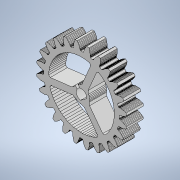
# Autodesk Inventor part: Деталь2
Saved by Autodesk Inventor 2020 (Build 240168000, 168)
## iProperties
Created: 2021-10-09
Part Number: Деталь2
Material: Типовые
Document SubType Name: Modeling
Designer: Антон
Density: 1 g/cm^3
Appearance: По умолчанию
Autodesk Inventor part; units mm, degrees
ref_plane "YZ Plane" through (0, 0, 0) normal (1, 0, 0) x (0, 1, 0)
ref_plane "XZ Plane" through (0, 0, 0) normal (0, 1, 0) x (-1, 0, 0)
ref_plane "XY Plane" through (0, 0, 0) normal (0, 0, 1) x (1, 0, 0)
sketch "a" plane through (0, 0, 0) normal (0, 0, 1) x (1, 0, 0)
  line L0 (2.444, 10.7729) -> (2.3647, 10.8798)
  line L1 (2.3647, 10.8798) -> (2.3022, 10.9131)
  line L2 (2.3022, 10.9131) -> (2.2426, 10.933)
  line L3 (2.2426, 10.933) -> (2.1279, 10.953)
  line L4 (2.1279, 10.953) -> (2.0158, 10.9612)
  line L5 (2.0158, 10.9612) -> (1.9071, 10.9524)
  line L6 (1.9071, 10.9524) -> (1.6861, 10.9538)
  line L7 (1.6861, 10.9538) -> (1.4617, 10.9732)
  line L8 (1.4617, 10.9732) -> (1.2349, 11.0072)
  line L9 (1.2349, 11.0072) -> (1.0063, 11.0542)
  line L10 (1.0063, 11.0542) -> (0.7762, 11.1131)
  line L11 (0.7762, 11.1131) -> (0.5451, 11.1834)
  line L12 (0.5451, 11.1834) -> (0.3132, 11.2645)
  line L13 (0.3132, 11.2645) -> (0.1389, 11.3323)
  line L14 (0.1389, 11.3323) -> (0.0609, 11.9767)
  line L15 (0.0609, 11.9767) -> (0.214, 12.084)
  line L16 (0.214, 12.084) -> (0.4199, 12.2181)
  line L17 (0.4199, 12.2181) -> (0.6276, 12.3415)
  line L18 (0.6276, 12.3415) -> (0.837, 12.4537)
  line L19 (0.837, 12.4537) -> (1.0478, 12.5538)
  line L20 (1.0478, 12.5538) -> (1.2599, 12.6409)
  line L21 (1.2599, 12.6409) -> (1.4731, 12.7133)
  line L22 (1.4731, 12.7133) -> (1.6875, 12.7674)
  line L23 (1.6875, 12.7674) -> (1.7951, 12.7847)
  line L24 (1.7951, 12.7847) -> (1.9021, 12.8194)
  line L25 (1.9021, 12.8194) -> (2.0087, 12.8663)
  line L26 (2.0087, 12.8663) -> (2.0617, 12.8998)
  line L27 (2.0617, 12.8998) -> (2.1145, 12.947)
  line L28 (2.1145, 12.947) -> (2.166, 13.0697)
  line L29 (2.166, 13.0697) -> (2.1721, 13.6527)
  line L30 (2.1721, 13.6527) -> (2.1232, 13.7765)
  line L31 (2.1232, 13.7765) -> (2.0714, 13.8248)
  line L32 (2.0714, 13.8248) -> (2.0191, 13.8595)
  line L33 (2.0191, 13.8595) -> (1.9135, 13.9085)
  line L34 (1.9135, 13.9085) -> (1.8073, 13.9455)
  line L35 (1.8073, 13.9455) -> (1.7, 13.965)
  line L36 (1.7, 13.965) -> (1.4869, 14.0236)
  line L37 (1.4869, 14.0236) -> (1.2752, 14.1004)
  line L38 (1.2752, 14.1004) -> (1.0649, 14.1919)
  line L39 (1.0649, 14.1919) -> (0.8563, 14.2965)
  line L40 (0.8563, 14.2965) -> (0.6493, 14.413)
  line L41 (0.6493, 14.413) -> (0.4442, 14.5407)
  line L42 (0.4442, 14.5407) -> (0.2412, 14.6791)
  line L43 (0.2412, 14.6791) -> (0.0903, 14.7897)
  line L44 (0.0903, 14.7897) -> (0.1818, 15.4322)
  line L45 (0.1818, 15.4322) -> (0.3575, 15.4963)
  line L46 (0.3575, 15.4963) -> (0.591, 15.5726)
  line L47 (0.591, 15.5726) -> (0.8236, 15.638)
  line L48 (0.8236, 15.638) -> (1.0549, 15.6921)
  line L49 (1.0549, 15.6921) -> (1.2845, 15.7343)
  line L50 (1.2845, 15.7343) -> (1.5119, 15.7636)
  line L51 (1.5119, 15.7636) -> (1.7366, 15.7782)
  line L52 (1.7366, 15.7782) -> (1.9576, 15.775)
  line L53 (1.9576, 15.775) -> (2.0661, 15.7639)
  line L54 (2.0661, 15.7639) -> (2.1784, 15.7697)
  line L55 (2.1784, 15.7697) -> (2.2935, 15.7874)
  line L56 (2.2935, 15.7874) -> (2.3534, 15.8061)
  line L57 (2.3534, 15.8061) -> (2.4166, 15.838)
  line L58 (2.4166, 15.838) -> (2.4981, 15.9432)
  line L59 (2.4981, 15.9432) -> (2.6549, 16.5048)
  line L60 (2.6549, 16.5048) -> (2.6397, 16.637)
  line L61 (2.6397, 16.637) -> (2.6022, 16.6971)
  line L62 (2.6022, 16.6971) -> (2.5606, 16.7441)
  line L63 (2.5606, 16.7441) -> (2.4713, 16.8188)
  line L64 (2.4713, 16.8188) -> (2.3782, 16.882)
  line L65 (2.3782, 16.882) -> (2.2797, 16.9286)
  line L66 (2.2797, 16.9286) -> (2.089, 17.0404)
  line L67 (2.089, 17.0404) -> (1.9044, 17.1693)
  line L68 (1.9044, 17.1693) -> (1.725, 17.3122)
  line L69 (1.725, 17.3122) -> (1.5505, 17.4672)
  line L70 (1.5505, 17.4672) -> (1.3807, 17.6333)
  line L71 (1.3807, 17.6333) -> (1.2157, 17.8097)
  line L72 (1.2157, 17.8097) -> (1.0554, 17.996)
  line L73 (1.0554, 17.996) -> (0.9383, 18.1418)
  line L74 (0.9383, 18.1418) -> (1.193, 18.7388)
  line L75 (1.193, 18.7388) -> (1.3792, 18.7552)
  line L76 (1.3792, 18.7552) -> (1.6246, 18.7684)
  line L77 (1.6246, 18.7684) -> (1.8662, 18.7714)
  line L78 (1.8662, 18.7714) -> (2.1036, 18.7639)
  line L79 (2.1036, 18.7639) -> (2.3362, 18.7452)
  line L80 (2.3362, 18.7452) -> (2.5635, 18.7146)
  line L81 (2.5635, 18.7146) -> (2.7843, 18.6706)
  line L82 (2.7843, 18.6706) -> (2.997, 18.6103)
  line L83 (2.997, 18.6103) -> (3.0989, 18.5715)
  line L84 (3.0989, 18.5715) -> (3.2088, 18.548)
  line L85 (3.2088, 18.548) -> (3.3246, 18.5353)
  line L86 (3.3246, 18.5353) -> (3.3873, 18.5378)
  line L87 (3.3873, 18.5378) -> (3.4566, 18.5523)
  line L88 (3.4566, 18.5523) -> (3.5626, 18.6328)
  line L89 (3.5626, 18.6328) -> (3.8594, 19.1347)
  line L90 (3.8594, 19.1347) -> (3.8789, 19.2664)
  line L91 (3.8789, 19.2664) -> (3.8582, 19.3341)
  line L92 (3.8582, 19.3341) -> (3.8302, 19.3902)
  line L93 (3.8302, 19.3902) -> (3.7633, 19.4855)
  line L94 (3.7633, 19.4855) -> (3.6898, 19.5707)
  line L95 (3.6898, 19.5707) -> (3.6067, 19.6412)
  line L96 (3.6067, 19.6412) -> (3.4514, 19.7985)
  line L97 (3.4514, 19.7985) -> (3.3065, 19.9709)
  line L98 (3.3065, 19.9709) -> (3.1701, 20.1552)
  line L99 (3.1701, 20.1552) -> (3.0417, 20.3501)
  line L100 (3.0417, 20.3501) -> (2.9207, 20.5545)
  line L101 (2.9207, 20.5545) -> (2.807, 20.7677)
  line L102 (2.807, 20.7677) -> (2.7003, 20.989)
  line L103 (2.7003, 20.989) -> (2.625, 21.1602)
  line L104 (2.625, 21.1602) -> (3.0255, 21.671)
  line L105 (3.0255, 21.671) -> (3.2096, 21.6386)
  line L106 (3.2096, 21.6386) -> (3.4501, 21.5878)
  line L107 (3.4501, 21.5878) -> (3.6842, 21.5282)
  line L108 (3.6842, 21.5282) -> (3.9115, 21.4595)
  line L109 (3.9115, 21.4595) -> (4.1314, 21.3812)
  line L110 (4.1314, 21.3812) -> (4.343, 21.2929)
  line L111 (4.343, 21.2929) -> (4.545, 21.1932)
  line L112 (4.545, 21.1932) -> (4.7348, 21.0799)
  line L113 (4.7348, 21.0799) -> (4.8231, 21.016)
  line L114 (4.8231, 21.016) -> (4.9233, 20.965)
  line L115 (4.9233, 20.965) -> (5.0318, 20.9227)
  line L116 (5.0318, 20.9227) -> (5.093, 20.9089)
  line L117 (5.093, 20.9089) -> (5.1637, 20.9049)
  line L118 (5.1637, 20.9049) -> (5.287, 20.9553)
  line L119 (5.287, 20.9553) -> (5.7035, 21.3632)
  line L120 (5.7035, 21.3632) -> (5.7565, 21.4854)
  line L121 (5.7565, 21.4854) -> (5.754, 21.5561)
  line L122 (5.754, 21.5561) -> (5.7415, 21.6176)
  line L123 (5.7415, 21.6176) -> (5.7015, 21.727)
  line L124 (5.7015, 21.727) -> (5.6525, 21.8283)
  line L125 (5.6525, 21.8283) -> (5.5905, 21.9179)
  line L126 (5.5905, 21.9179) -> (5.4812, 22.1101)
  line L127 (5.4812, 22.1101) -> (5.3858, 22.314)
  line L128 (5.3858, 22.314) -> (5.3019, 22.5274)
  line L129 (5.3019, 22.5274) -> (5.2283, 22.7489)
  line L130 (5.2283, 22.7489) -> (5.1643, 22.9777)
  line L131 (5.1643, 22.9777) -> (5.1096, 23.213)
  line L132 (5.1096, 23.213) -> (5.0639, 23.4544)
  line L133 (5.0639, 23.4544) -> (5.0354, 23.6392)
  line L134 (5.0354, 23.6392) -> (5.5544, 24.0289)
  line L135 (5.5544, 24.0289) -> (5.724, 23.95)
  line L136 (5.724, 23.95) -> (5.943, 23.8388)
  line L137 (5.943, 23.8388) -> (6.1538, 23.7206)
  line L138 (6.1538, 23.7206) -> (6.3556, 23.5953)
  line L139 (6.3556, 23.5953) -> (6.5477, 23.4628)
  line L140 (6.5477, 23.4628) -> (6.7292, 23.3227)
  line L141 (6.7292, 23.3227) -> (6.8985, 23.1742)
  line L142 (6.8985, 23.1742) -> (7.0525, 23.0156)
  line L143 (7.0525, 23.0156) -> (7.1213, 22.9311)
  line L144 (7.1213, 22.9311) -> (7.2049, 22.8558)
  line L145 (7.2049, 22.8558) -> (7.2988, 22.7869)
  line L146 (7.2988, 22.7869) -> (7.3543, 22.7577)
  line L147 (7.3543, 22.7577) -> (7.4216, 22.7356)
  line L148 (7.4216, 22.7356) -> (7.5536, 22.7523)
  line L149 (7.5536, 22.7523) -> (8.0616, 23.0386)
  line L150 (8.0616, 23.0386) -> (8.1443, 23.1428)
  line L151 (8.1443, 23.1428) -> (8.1603, 23.2118)
  line L152 (8.1603, 23.2118) -> (8.1641, 23.2745)
  line L153 (8.1641, 23.2745) -> (8.1538, 23.3905)
  line L154 (8.1538, 23.3905) -> (8.1327, 23.5009)
  line L155 (8.1327, 23.5009) -> (8.096, 23.6036)
  line L156 (8.096, 23.6036) -> (8.0402, 23.8175)
  line L157 (8.0402, 23.8175) -> (8.0008, 24.0392)
  line L158 (8.0008, 24.0392) -> (7.975, 24.267)
  line L159 (7.975, 24.267) -> (7.9612, 24.5)
  line L160 (7.9612, 24.5) -> (7.9586, 24.7375)
  line L161 (7.9586, 24.7375) -> (7.9666, 24.979)
  line L162 (7.9666, 24.979) -> (7.985, 25.224)
  line L163 (7.985, 25.224) -> (8.0053, 25.4099)
  line L164 (8.0053, 25.4099) -> (8.6075, 25.652)
  line L165 (8.6075, 25.652) -> (8.7508, 25.5319)
  line L166 (8.7508, 25.5319) -> (8.9337, 25.3677)
  line L167 (8.9337, 25.3677) -> (9.1066, 25.199)
  line L168 (9.1066, 25.199) -> (9.2691, 25.0258)
  line L169 (9.2691, 25.0258) -> (9.4205, 24.8481)
  line L170 (9.4205, 24.8481) -> (9.5595, 24.6658)
  line L171 (9.5595, 24.6658) -> (9.6846, 24.4785)
  line L172 (9.6846, 24.4785) -> (9.7923, 24.2855)
  line L173 (9.7923, 24.2855) -> (9.8369, 24.186)
  line L174 (9.8369, 24.186) -> (9.8981, 24.0917)
  line L175 (9.8981, 24.0917) -> (9.9709, 24.0008)
  line L176 (9.9709, 24.0008) -> (10.0171, 23.9582)
  line L177 (10.0171, 23.9582) -> (10.0763, 23.9195)
  line L178 (10.0763, 23.9195) -> (10.2082, 23.9015)
  line L179 (10.2082, 23.9015) -> (10.7729, 24.0465)
  line L180 (10.7729, 24.0465) -> (10.8798, 24.1258)
  line L181 (10.8798, 24.1258) -> (10.9131, 24.1883)
  line L182 (10.9131, 24.1883) -> (10.933, 24.2478)
  line L183 (10.933, 24.2478) -> (10.953, 24.3626)
  line L184 (10.953, 24.3626) -> (10.9612, 24.4747)
  line L185 (10.9612, 24.4747) -> (10.9524, 24.5833)
  line L186 (10.9524, 24.5833) -> (10.9538, 24.8044)
  line L187 (10.9538, 24.8044) -> (10.9732, 25.0287)
  line L188 (10.9732, 25.0287) -> (11.0072, 25.2555)
  line L189 (11.0072, 25.2555) -> (11.0542, 25.4842)
  line L190 (11.0542, 25.4842) -> (11.1131, 25.7142)
  line L191 (11.1131, 25.7142) -> (11.1834, 25.9454)
  line L192 (11.1834, 25.9454) -> (11.2645, 26.1773)
  line L193 (11.2645, 26.1773) -> (11.3323, 26.3516)
  line L194 (11.3323, 26.3516) -> (11.9767, 26.4296)
  line L195 (11.9767, 26.4296) -> (12.084, 26.2765)
  line L196 (12.084, 26.2765) -> (12.2181, 26.0706)
  line L197 (12.2181, 26.0706) -> (12.3415, 25.8629)
  line L198 (12.3415, 25.8629) -> (12.4537, 25.6535)
  line L199 (12.4537, 25.6535) -> (12.5538, 25.4427)
  line L200 (12.5538, 25.4427) -> (12.6409, 25.2306)
  line L201 (12.6409, 25.2306) -> (12.7133, 25.0173)
  line L202 (12.7133, 25.0173) -> (12.7674, 24.803)
  line L203 (12.7674, 24.803) -> (12.7847, 24.6954)
  line L204 (12.7847, 24.6954) -> (12.8194, 24.5884)
  line L205 (12.8194, 24.5884) -> (12.8663, 24.4818)
  line L206 (12.8663, 24.4818) -> (12.8998, 24.4287)
  line L207 (12.8998, 24.4287) -> (12.947, 24.3759)
  line L208 (12.947, 24.3759) -> (13.0697, 24.3244)
  line L209 (13.0697, 24.3244) -> (13.6527, 24.3183)
  line L210 (13.6527, 24.3183) -> (13.7765, 24.3673)
  line L211 (13.7765, 24.3673) -> (13.8248, 24.419)
  line L212 (13.8248, 24.419) -> (13.8595, 24.4714)
  line L213 (13.8595, 24.4714) -> (13.9085, 24.577)
  line L214 (13.9085, 24.577) -> (13.9455, 24.6832)
  line L215 (13.9455, 24.6832) -> (13.965, 24.7904)
  line L216 (13.965, 24.7904) -> (14.0236, 25.0036)
  line L217 (14.0236, 25.0036) -> (14.1004, 25.2153)
  line L218 (14.1004, 25.2153) -> (14.1919, 25.4255)
  line L219 (14.1919, 25.4255) -> (14.2965, 25.6342)
  line L220 (14.2965, 25.6342) -> (14.413, 25.8412)
  line L221 (14.413, 25.8412) -> (14.5407, 26.0463)
  line L222 (14.5407, 26.0463) -> (14.6791, 26.2493)
  line L223 (14.6791, 26.2493) -> (14.7897, 26.4001)
  line L224 (14.7897, 26.4001) -> (15.4322, 26.3087)
  line L225 (15.4322, 26.3087) -> (15.4963, 26.133)
  line L226 (15.4963, 26.133) -> (15.5726, 25.8994)
  line L227 (15.5726, 25.8994) -> (15.638, 25.6668)
  line L228 (15.638, 25.6668) -> (15.6921, 25.4356)
  line L229 (15.6921, 25.4356) -> (15.7343, 25.206)
  line L230 (15.7343, 25.206) -> (15.7636, 24.9786)
  line L231 (15.7636, 24.9786) -> (15.7782, 24.7539)
  line L232 (15.7782, 24.7539) -> (15.775, 24.5329)
  line L233 (15.775, 24.5329) -> (15.7639, 24.4244)
  line L234 (15.7639, 24.4244) -> (15.7697, 24.3121)
  line L235 (15.7697, 24.3121) -> (15.7874, 24.197)
  line L236 (15.7874, 24.197) -> (15.8061, 24.1371)
  line L237 (15.8061, 24.1371) -> (15.838, 24.0739)
  line L238 (15.838, 24.0739) -> (15.9432, 23.9924)
  line L239 (15.9432, 23.9924) -> (16.5048, 23.8356)
  line L240 (16.5048, 23.8356) -> (16.637, 23.8508)
  line L241 (16.637, 23.8508) -> (16.6971, 23.8883)
  line L242 (16.6971, 23.8883) -> (16.7441, 23.9299)
  line L243 (16.7441, 23.9299) -> (16.8188, 24.0192)
  line L244 (16.8188, 24.0192) -> (16.882, 24.1122)
  line L245 (16.882, 24.1122) -> (16.9286, 24.2108)
  line L246 (16.9286, 24.2108) -> (17.0404, 24.4015)
  line L247 (17.0404, 24.4015) -> (17.1693, 24.5861)
  line L248 (17.1693, 24.5861) -> (17.3122, 24.7655)
  line L249 (17.3122, 24.7655) -> (17.4672, 24.94)
  line L250 (17.4672, 24.94) -> (17.6333, 25.1097)
  line L251 (17.6333, 25.1097) -> (17.8097, 25.2748)
  line L252 (17.8097, 25.2748) -> (17.996, 25.4351)
  line L253 (17.996, 25.4351) -> (18.1418, 25.5522)
  line L254 (18.1418, 25.5522) -> (18.7388, 25.2975)
  line L255 (18.7388, 25.2975) -> (18.7552, 25.1112)
  line L256 (18.7552, 25.1112) -> (18.7684, 24.8659)
  line L257 (18.7684, 24.8659) -> (18.7714, 24.6243)
  line L258 (18.7714, 24.6243) -> (18.7639, 24.3869)
  line L259 (18.7639, 24.3869) -> (18.7452, 24.1542)
  line L260 (18.7452, 24.1542) -> (18.7146, 23.927)
  line L261 (18.7146, 23.927) -> (18.6706, 23.7061)
  line L262 (18.6706, 23.7061) -> (18.6103, 23.4935)
  line L263 (18.6103, 23.4935) -> (18.5715, 23.3916)
  line L264 (18.5715, 23.3916) -> (18.548, 23.2816)
  line L265 (18.548, 23.2816) -> (18.5353, 23.1659)
  line L266 (18.5353, 23.1659) -> (18.5378, 23.1031)
  line L267 (18.5378, 23.1031) -> (18.5523, 23.0338)
  line L268 (18.5523, 23.0338) -> (18.6328, 22.9279)
  line L269 (18.6328, 22.9279) -> (19.1347, 22.6311)
  line L270 (19.1347, 22.6311) -> (19.2664, 22.6115)
  line L271 (19.2664, 22.6115) -> (19.3341, 22.6322)
  line L272 (19.3341, 22.6322) -> (19.3902, 22.6603)
  line L273 (19.3902, 22.6603) -> (19.4855, 22.7272)
  line L274 (19.4855, 22.7272) -> (19.5707, 22.8007)
  line L275 (19.5707, 22.8007) -> (19.6412, 22.8838)
  line L276 (19.6412, 22.8838) -> (19.7985, 23.0391)
  line L277 (19.7985, 23.0391) -> (19.9709, 23.184)
  line L278 (19.9709, 23.184) -> (20.1552, 23.3203)
  line L279 (20.1552, 23.3203) -> (20.3501, 23.4488)
  line L280 (20.3501, 23.4488) -> (20.5545, 23.5698)
  line L281 (20.5545, 23.5698) -> (20.7677, 23.6835)
  line L282 (20.7677, 23.6835) -> (20.989, 23.7902)
  line L283 (20.989, 23.7902) -> (21.1602, 23.8655)
  line L284 (21.1602, 23.8655) -> (21.671, 23.465)
  line L285 (21.671, 23.465) -> (21.6386, 23.2808)
  line L286 (21.6386, 23.2808) -> (21.5878, 23.0404)
  line L287 (21.5878, 23.0404) -> (21.5282, 22.8063)
  line L288 (21.5282, 22.8063) -> (21.4595, 22.5789)
  line L289 (21.4595, 22.5789) -> (21.3812, 22.359)
  line L290 (21.3812, 22.359) -> (21.2929, 22.1475)
  line L291 (21.2929, 22.1475) -> (21.1932, 21.9455)
  line L292 (21.1932, 21.9455) -> (21.0799, 21.7557)
  line L293 (21.0799, 21.7557) -> (21.016, 21.6674)
  line L294 (21.016, 21.6674) -> (20.965, 21.5672)
  line L295 (20.965, 21.5672) -> (20.9227, 21.4587)
  line L296 (20.9227, 21.4587) -> (20.9089, 21.3974)
  line L297 (20.9089, 21.3974) -> (20.9049, 21.3267)
  line L298 (20.9049, 21.3267) -> (20.9553, 21.2035)
  line L299 (20.9553, 21.2035) -> (21.3632, 20.7869)
  line L300 (21.3632, 20.7869) -> (21.4854, 20.734)
  line L301 (21.4854, 20.734) -> (21.5561, 20.7365)
  line L302 (21.5561, 20.7365) -> (21.6176, 20.749)
  line L303 (21.6176, 20.749) -> (21.727, 20.789)
  line L304 (21.727, 20.789) -> (21.8283, 20.838)
  line L305 (21.8283, 20.838) -> (21.9179, 20.9)
  line L306 (21.9179, 20.9) -> (22.1101, 21.0093)
  line L307 (22.1101, 21.0093) -> (22.314, 21.1046)
  line L308 (22.314, 21.1046) -> (22.5274, 21.1886)
  line L309 (22.5274, 21.1886) -> (22.7489, 21.2622)
  line L310 (22.7489, 21.2622) -> (22.9777, 21.3262)
  line L311 (22.9777, 21.3262) -> (23.213, 21.3809)
  line L312 (23.213, 21.3809) -> (23.4544, 21.4266)
  line L313 (23.4544, 21.4266) -> (23.6392, 21.4551)
  line L314 (23.6392, 21.4551) -> (24.0289, 20.936)
  line L315 (24.0289, 20.936) -> (23.95, 20.7665)
  line L316 (23.95, 20.7665) -> (23.8388, 20.5474)
  line L317 (23.8388, 20.5474) -> (23.7206, 20.3367)
  line L318 (23.7206, 20.3367) -> (23.5953, 20.1349)
  line L319 (23.5953, 20.1349) -> (23.4628, 19.9427)
  line L320 (23.4628, 19.9427) -> (23.3227, 19.7612)
  line L321 (23.3227, 19.7612) -> (23.1742, 19.592)
  line L322 (23.1742, 19.592) -> (23.0156, 19.4379)
  line L323 (23.0156, 19.4379) -> (22.9311, 19.3692)
  line L324 (22.9311, 19.3692) -> (22.8558, 19.2856)
  line L325 (22.8558, 19.2856) -> (22.7869, 19.1917)
  line L326 (22.7869, 19.1917) -> (22.7577, 19.1361)
  line L327 (22.7577, 19.1361) -> (22.7356, 19.0689)
  line L328 (22.7356, 19.0689) -> (22.7523, 18.9368)
  line L329 (22.7523, 18.9368) -> (23.0386, 18.4289)
  line L330 (23.0386, 18.4289) -> (23.1428, 18.3461)
  line L331 (23.1428, 18.3461) -> (23.2118, 18.3302)
  line L332 (23.2118, 18.3302) -> (23.2745, 18.3264)
  line L333 (23.2745, 18.3264) -> (23.3905, 18.3367)
  line L334 (23.3905, 18.3367) -> (23.5009, 18.3578)
  line L335 (23.5009, 18.3578) -> (23.6036, 18.3945)
  line L336 (23.6036, 18.3945) -> (23.8175, 18.4503)
  line L337 (23.8175, 18.4503) -> (24.0392, 18.4897)
  line L338 (24.0392, 18.4897) -> (24.267, 18.5155)
  line L339 (24.267, 18.5155) -> (24.5, 18.5293)
  line L340 (24.5, 18.5293) -> (24.7375, 18.5319)
  line L341 (24.7375, 18.5319) -> (24.979, 18.5238)
  line L342 (24.979, 18.5238) -> (25.224, 18.5055)
  line L343 (25.224, 18.5055) -> (25.4099, 18.4852)
  line L344 (25.4099, 18.4852) -> (25.652, 17.883)
  line L345 (25.652, 17.883) -> (25.5319, 17.7396)
  line L346 (25.5319, 17.7396) -> (25.3677, 17.5568)
  line L347 (25.3677, 17.5568) -> (25.199, 17.3839)
  line L348 (25.199, 17.3839) -> (25.0258, 17.2213)
  line L349 (25.0258, 17.2213) -> (24.8481, 17.07)
  line L350 (24.8481, 17.07) -> (24.6658, 16.931)
  line L351 (24.6658, 16.931) -> (24.4785, 16.8059)
  line L352 (24.4785, 16.8059) -> (24.2855, 16.6982)
  line L353 (24.2855, 16.6982) -> (24.186, 16.6536)
  line L354 (24.186, 16.6536) -> (24.0917, 16.5924)
  line L355 (24.0917, 16.5924) -> (24.0008, 16.5195)
  line L356 (24.0008, 16.5195) -> (23.9582, 16.4734)
  line L357 (23.9582, 16.4734) -> (23.9195, 16.4142)
  line L358 (23.9195, 16.4142) -> (23.9015, 16.2823)
  line L359 (23.9015, 16.2823) -> (24.0465, 15.7175)
  line L360 (24.0465, 15.7175) -> (24.1258, 15.6106)
  line L361 (24.1258, 15.6106) -> (24.1883, 15.5774)
  line L362 (24.1883, 15.5774) -> (24.2478, 15.5575)
  line L363 (24.2478, 15.5575) -> (24.3626, 15.5374)
  line L364 (24.3626, 15.5374) -> (24.4747, 15.5292)
  line L365 (24.4747, 15.5292) -> (24.5833, 15.5381)
  line L366 (24.5833, 15.5381) -> (24.8044, 15.5367)
  line L367 (24.8044, 15.5367) -> (25.0287, 15.5173)
  line L368 (25.0287, 15.5173) -> (25.2555, 15.4833)
  line L369 (25.2555, 15.4833) -> (25.4842, 15.4363)
  line L370 (25.4842, 15.4363) -> (25.7142, 15.3773)
  line L371 (25.7142, 15.3773) -> (25.9454, 15.307)
  line L372 (25.9454, 15.307) -> (26.1773, 15.2259)
  line L373 (26.1773, 15.2259) -> (26.3516, 15.1582)
  line L374 (26.3516, 15.1582) -> (26.4296, 14.5138)
  line L375 (26.4296, 14.5138) -> (26.2765, 14.4065)
  line L376 (26.2765, 14.4065) -> (26.0706, 14.2724)
  line L377 (26.0706, 14.2724) -> (25.8629, 14.149)
  line L378 (25.8629, 14.149) -> (25.6535, 14.0368)
  line L379 (25.6535, 14.0368) -> (25.4427, 13.9366)
  line L380 (25.4427, 13.9366) -> (25.2306, 13.8495)
  line L381 (25.2306, 13.8495) -> (25.0173, 13.7772)
  line L382 (25.0173, 13.7772) -> (24.803, 13.7231)
  line L383 (24.803, 13.7231) -> (24.6954, 13.7058)
  line L384 (24.6954, 13.7058) -> (24.5884, 13.6711)
  line L385 (24.5884, 13.6711) -> (24.4818, 13.6242)
  line L386 (24.4818, 13.6242) -> (24.4287, 13.5907)
  line L387 (24.4287, 13.5907) -> (24.3759, 13.5435)
  line L388 (24.3759, 13.5435) -> (24.3244, 13.4208)
  line L389 (24.3244, 13.4208) -> (24.3183, 12.8377)
  line L390 (24.3183, 12.8377) -> (24.3673, 12.7139)
  line L391 (24.3673, 12.7139) -> (24.419, 12.6657)
  line L392 (24.419, 12.6657) -> (24.4714, 12.631)
  line L393 (24.4714, 12.631) -> (24.577, 12.5819)
  line L394 (24.577, 12.5819) -> (24.6832, 12.545)
  line L395 (24.6832, 12.545) -> (24.7904, 12.5254)
  line L396 (24.7904, 12.5254) -> (25.0036, 12.4669)
  line L397 (25.0036, 12.4669) -> (25.2153, 12.3901)
  line L398 (25.2153, 12.3901) -> (25.4255, 12.2985)
  line L399 (25.4255, 12.2985) -> (25.6342, 12.194)
  line L400 (25.6342, 12.194) -> (25.8412, 12.0775)
  line L401 (25.8412, 12.0775) -> (26.0463, 11.9498)
  line L402 (26.0463, 11.9498) -> (26.2493, 11.8114)
  line L403 (26.2493, 11.8114) -> (26.4001, 11.7008)
  line L404 (26.4001, 11.7008) -> (26.3087, 11.0582)
  line L405 (26.3087, 11.0582) -> (26.133, 10.9942)
  line L406 (26.133, 10.9942) -> (25.8994, 10.9179)
  line L407 (25.8994, 10.9179) -> (25.6668, 10.8525)
  line L408 (25.6668, 10.8525) -> (25.4356, 10.7983)
  line L409 (25.4356, 10.7983) -> (25.206, 10.7561)
  line L410 (25.206, 10.7561) -> (24.9786, 10.7269)
  line L411 (24.9786, 10.7269) -> (24.7539, 10.7122)
  line L412 (24.7539, 10.7122) -> (24.5329, 10.7154)
  line L413 (24.5329, 10.7154) -> (24.4244, 10.7266)
  line L414 (24.4244, 10.7266) -> (24.3121, 10.7207)
  line L415 (24.3121, 10.7207) -> (24.197, 10.7031)
  line L416 (24.197, 10.7031) -> (24.1371, 10.6844)
  line L417 (24.1371, 10.6844) -> (24.0739, 10.6525)
  line L418 (24.0739, 10.6525) -> (23.9924, 10.5473)
  line L419 (23.9924, 10.5473) -> (23.8356, 9.9857)
  line L420 (23.8356, 9.9857) -> (23.8508, 9.8535)
  line L421 (23.8508, 9.8535) -> (23.8883, 9.7934)
  line L422 (23.8883, 9.7934) -> (23.9299, 9.7464)
  line L423 (23.9299, 9.7464) -> (24.0192, 9.6717)
  line L424 (24.0192, 9.6717) -> (24.1122, 9.6085)
  line L425 (24.1122, 9.6085) -> (24.2108, 9.5618)
  line L426 (24.2108, 9.5618) -> (24.4015, 9.4501)
  line L427 (24.4015, 9.4501) -> (24.5861, 9.3211)
  line L428 (24.5861, 9.3211) -> (24.7655, 9.1783)
  line L429 (24.7655, 9.1783) -> (24.94, 9.0233)
  line L430 (24.94, 9.0233) -> (25.1097, 8.8572)
  line L431 (25.1097, 8.8572) -> (25.2748, 8.6807)
  line L432 (25.2748, 8.6807) -> (25.4351, 8.4945)
  line L433 (25.4351, 8.4945) -> (25.5522, 8.3487)
  line L434 (25.5522, 8.3487) -> (25.2975, 7.7517)
  line L435 (25.2975, 7.7517) -> (25.1112, 7.7353)
  line L436 (25.1112, 7.7353) -> (24.8659, 7.7221)
  line L437 (24.8659, 7.7221) -> (24.6243, 7.7191)
  line L438 (24.6243, 7.7191) -> (24.3869, 7.7266)
  line L439 (24.3869, 7.7266) -> (24.1542, 7.7453)
  line L440 (24.1542, 7.7453) -> (23.927, 7.7759)
  line L441 (23.927, 7.7759) -> (23.7061, 7.8199)
  line L442 (23.7061, 7.8199) -> (23.4935, 7.8802)
  line L443 (23.4935, 7.8802) -> (23.3916, 7.919)
  line L444 (23.3916, 7.919) -> (23.2816, 7.9424)
  line L445 (23.2816, 7.9424) -> (23.1659, 7.9552)
  line L446 (23.1659, 7.9552) -> (23.1031, 7.9527)
  line L447 (23.1031, 7.9527) -> (23.0338, 7.9382)
  line L448 (23.0338, 7.9382) -> (22.9279, 7.8576)
  line L449 (22.9279, 7.8576) -> (22.6311, 7.3558)
  line L450 (22.6311, 7.3558) -> (22.6115, 7.2241)
  line L451 (22.6115, 7.2241) -> (22.6322, 7.1564)
  line L452 (22.6322, 7.1564) -> (22.6603, 7.1002)
  line L453 (22.6603, 7.1002) -> (22.7272, 7.0049)
  line L454 (22.7272, 7.0049) -> (22.8007, 6.9198)
  line L455 (22.8007, 6.9198) -> (22.8838, 6.8493)
  line L456 (22.8838, 6.8493) -> (23.0391, 6.692)
  line L457 (23.0391, 6.692) -> (23.184, 6.5196)
  line L458 (23.184, 6.5196) -> (23.3203, 6.3352)
  line L459 (23.3203, 6.3352) -> (23.4488, 6.1403)
  line L460 (23.4488, 6.1403) -> (23.5698, 5.936)
  line L461 (23.5698, 5.936) -> (23.6835, 5.7228)
  line L462 (23.6835, 5.7228) -> (23.7902, 5.5014)
  line L463 (23.7902, 5.5014) -> (23.8655, 5.3303)
  line L464 (23.8655, 5.3303) -> (23.465, 4.8195)
  line L465 (23.465, 4.8195) -> (23.2808, 4.8519)
  line L466 (23.2808, 4.8519) -> (23.0404, 4.9026)
  line L467 (23.0404, 4.9026) -> (22.8063, 4.9623)
  line L468 (22.8063, 4.9623) -> (22.5789, 5.031)
  line L469 (22.5789, 5.031) -> (22.359, 5.1092)
  line L470 (22.359, 5.1092) -> (22.1475, 5.1976)
  line L471 (22.1475, 5.1976) -> (21.9455, 5.2973)
  line L472 (21.9455, 5.2973) -> (21.7557, 5.4105)
  line L473 (21.7557, 5.4105) -> (21.6674, 5.4744)
  line L474 (21.6674, 5.4744) -> (21.5672, 5.5255)
  line L475 (21.5672, 5.5255) -> (21.4587, 5.5678)
  line L476 (21.4587, 5.5678) -> (21.3974, 5.5816)
  line L477 (21.3974, 5.5816) -> (21.3267, 5.5855)
  line L478 (21.3267, 5.5855) -> (21.2035, 5.5352)
  line L479 (21.2035, 5.5352) -> (20.7869, 5.1272)
  line L480 (20.7869, 5.1272) -> (20.734, 5.0051)
  line L481 (20.734, 5.0051) -> (20.7365, 4.9343)
  line L482 (20.7365, 4.9343) -> (20.749, 4.8728)
  line L483 (20.749, 4.8728) -> (20.789, 4.7634)
  line L484 (20.789, 4.7634) -> (20.838, 4.6622)
  line L485 (20.838, 4.6622) -> (20.9, 4.5726)
  line L486 (20.9, 4.5726) -> (21.0093, 4.3804)
  line L487 (21.0093, 4.3804) -> (21.1046, 4.1764)
  line L488 (21.1046, 4.1764) -> (21.1886, 3.963)
  line L489 (21.1886, 3.963) -> (21.2622, 3.7416)
  line L490 (21.2622, 3.7416) -> (21.3262, 3.5128)
  line L491 (21.3262, 3.5128) -> (21.3809, 3.2775)
  line L492 (21.3809, 3.2775) -> (21.4266, 3.0361)
  line L493 (21.4266, 3.0361) -> (21.4551, 2.8513)
  line L494 (21.4551, 2.8513) -> (20.936, 2.4615)
  line L495 (20.936, 2.4615) -> (20.7665, 2.5405)
  line L496 (20.7665, 2.5405) -> (20.5474, 2.6517)
  line L497 (20.5474, 2.6517) -> (20.3367, 2.7699)
  line L498 (20.3367, 2.7699) -> (20.1349, 2.8951)
  line L499 (20.1349, 2.8951) -> (19.9427, 3.0276)
  line L500 (19.9427, 3.0276) -> (19.7612, 3.1678)
  line L501 (19.7612, 3.1678) -> (19.592, 3.3163)
  line L502 (19.592, 3.3163) -> (19.4379, 3.4749)
  line L503 (19.4379, 3.4749) -> (19.3692, 3.5594)
  line L504 (19.3692, 3.5594) -> (19.2856, 3.6347)
  line L505 (19.2856, 3.6347) -> (19.1917, 3.7036)
  line L506 (19.1917, 3.7036) -> (19.1361, 3.7328)
  line L507 (19.1361, 3.7328) -> (19.0689, 3.7549)
  line L508 (19.0689, 3.7549) -> (18.9368, 3.7381)
  line L509 (18.9368, 3.7381) -> (18.4289, 3.4519)
  line L510 (18.4289, 3.4519) -> (18.3461, 3.3476)
  line L511 (18.3461, 3.3476) -> (18.3302, 3.2787)
  line L512 (18.3302, 3.2787) -> (18.3264, 3.216)
  line L513 (18.3264, 3.216) -> (18.3367, 3.1)
  line L514 (18.3367, 3.1) -> (18.3578, 2.9895)
  line L515 (18.3578, 2.9895) -> (18.3945, 2.8869)
  line L516 (18.3945, 2.8869) -> (18.4503, 2.673)
  line L517 (18.4503, 2.673) -> (18.4897, 2.4513)
  line L518 (18.4897, 2.4513) -> (18.5155, 2.2234)
  line L519 (18.5155, 2.2234) -> (18.5293, 1.9904)
  line L520 (18.5293, 1.9904) -> (18.5319, 1.753)
  line L521 (18.5319, 1.753) -> (18.5238, 1.5115)
  line L522 (18.5238, 1.5115) -> (18.5055, 1.2664)
  line L523 (18.5055, 1.2664) -> (18.4852, 1.0806)
  line L524 (18.4852, 1.0806) -> (17.883, 0.8385)
  line L525 (17.883, 0.8385) -> (17.7396, 0.9586)
  line L526 (17.7396, 0.9586) -> (17.5568, 1.1227)
  line L527 (17.5568, 1.1227) -> (17.3839, 1.2914)
  line L528 (17.3839, 1.2914) -> (17.2213, 1.4646)
  line L529 (17.2213, 1.4646) -> (17.07, 1.6424)
  line L530 (17.07, 1.6424) -> (16.931, 1.8247)
  line L531 (16.931, 1.8247) -> (16.8059, 2.012)
  line L532 (16.8059, 2.012) -> (16.6982, 2.205)
  line L533 (16.6982, 2.205) -> (16.6536, 2.3045)
  line L534 (16.6536, 2.3045) -> (16.5924, 2.3988)
  line L535 (16.5924, 2.3988) -> (16.5195, 2.4897)
  line L536 (16.5195, 2.4897) -> (16.4734, 2.5322)
  line L537 (16.4734, 2.5322) -> (16.4142, 2.571)
  line L538 (16.4142, 2.571) -> (16.2823, 2.589)
  line L539 (16.2823, 2.589) -> (15.7175, 2.444)
  line L540 (15.7175, 2.444) -> (15.6106, 2.3647)
  line L541 (15.6106, 2.3647) -> (15.5774, 2.3022)
  line L542 (15.5774, 2.3022) -> (15.5575, 2.2426)
  line L543 (15.5575, 2.2426) -> (15.5374, 2.1279)
  line L544 (15.5374, 2.1279) -> (15.5292, 2.0158)
  line L545 (15.5292, 2.0158) -> (15.5381, 1.9071)
  line L546 (15.5381, 1.9071) -> (15.5367, 1.6861)
  line L547 (15.5367, 1.6861) -> (15.5173, 1.4617)
  line L548 (15.5173, 1.4617) -> (15.4833, 1.2349)
  line L549 (15.4833, 1.2349) -> (15.4363, 1.0063)
  line L550 (15.4363, 1.0063) -> (15.3773, 0.7762)
  line L551 (15.3773, 0.7762) -> (15.307, 0.5451)
  line L552 (15.307, 0.5451) -> (15.2259, 0.3132)
  line L553 (15.2259, 0.3132) -> (15.1582, 0.1389)
  line L554 (15.1582, 0.1389) -> (14.5138, 0.0609)
  line L555 (14.5138, 0.0609) -> (14.4065, 0.214)
  line L556 (14.4065, 0.214) -> (14.2724, 0.4199)
  line L557 (14.2724, 0.4199) -> (14.149, 0.6276)
  line L558 (14.149, 0.6276) -> (14.0368, 0.837)
  line L559 (14.0368, 0.837) -> (13.9366, 1.0478)
  line L560 (13.9366, 1.0478) -> (13.8495, 1.2599)
  line L561 (13.8495, 1.2599) -> (13.7772, 1.4731)
  line L562 (13.7772, 1.4731) -> (13.7231, 1.6875)
  line L563 (13.7231, 1.6875) -> (13.7058, 1.7951)
  line L564 (13.7058, 1.7951) -> (13.6711, 1.9021)
  line L565 (13.6711, 1.9021) -> (13.6242, 2.0087)
  line L566 (13.6242, 2.0087) -> (13.5907, 2.0617)
  line L567 (13.5907, 2.0617) -> (13.5435, 2.1145)
  line L568 (13.5435, 2.1145) -> (13.4208, 2.166)
  line L569 (13.4208, 2.166) -> (12.8377, 2.1721)
  line L570 (12.8377, 2.1721) -> (12.7139, 2.1232)
  line L571 (12.7139, 2.1232) -> (12.6657, 2.0714)
  line L572 (12.6657, 2.0714) -> (12.631, 2.0191)
  line L573 (12.631, 2.0191) -> (12.5819, 1.9135)
  line L574 (12.5819, 1.9135) -> (12.545, 1.8073)
  line L575 (12.545, 1.8073) -> (12.5254, 1.7)
  line L576 (12.5254, 1.7) -> (12.4669, 1.4869)
  line L577 (12.4669, 1.4869) -> (12.3901, 1.2752)
  line L578 (12.3901, 1.2752) -> (12.2985, 1.0649)
  line L579 (12.2985, 1.0649) -> (12.194, 0.8563)
  line L580 (12.194, 0.8563) -> (12.0775, 0.6493)
  line L581 (12.0775, 0.6493) -> (11.9498, 0.4442)
  line L582 (11.9498, 0.4442) -> (11.8114, 0.2412)
  line L583 (11.8114, 0.2412) -> (11.7008, 0.0903)
  line L584 (11.7008, 0.0903) -> (11.0582, 0.1818)
  line L585 (11.0582, 0.1818) -> (10.9942, 0.3575)
  line L586 (10.9942, 0.3575) -> (10.9179, 0.591)
  line L587 (10.9179, 0.591) -> (10.8525, 0.8236)
  line L588 (10.8525, 0.8236) -> (10.7983, 1.0549)
  line L589 (10.7983, 1.0549) -> (10.7561, 1.2845)
  line L590 (10.7561, 1.2845) -> (10.7269, 1.5119)
  line L591 (10.7269, 1.5119) -> (10.7122, 1.7366)
  line L592 (10.7122, 1.7366) -> (10.7154, 1.9576)
  line L593 (10.7154, 1.9576) -> (10.7266, 2.0661)
  line L594 (10.7266, 2.0661) -> (10.7207, 2.1784)
  line L595 (10.7207, 2.1784) -> (10.7031, 2.2935)
  line L596 (10.7031, 2.2935) -> (10.6844, 2.3534)
  line L597 (10.6844, 2.3534) -> (10.6525, 2.4166)
  line L598 (10.6525, 2.4166) -> (10.5473, 2.4981)
  line L599 (10.5473, 2.4981) -> (9.9857, 2.6549)
  line L600 (9.9857, 2.6549) -> (9.8535, 2.6397)
  line L601 (9.8535, 2.6397) -> (9.7934, 2.6022)
  line L602 (9.7934, 2.6022) -> (9.7464, 2.5606)
  line L603 (9.7464, 2.5606) -> (9.6717, 2.4713)
  line L604 (9.6717, 2.4713) -> (9.6085, 2.3782)
  line L605 (9.6085, 2.3782) -> (9.5618, 2.2797)
  line L606 (9.5618, 2.2797) -> (9.4501, 2.089)
  line L607 (9.4501, 2.089) -> (9.3211, 1.9044)
  line L608 (9.3211, 1.9044) -> (9.1783, 1.725)
  line L609 (9.1783, 1.725) -> (9.0233, 1.5505)
  line L610 (9.0233, 1.5505) -> (8.8572, 1.3807)
  line L611 (8.8572, 1.3807) -> (8.6807, 1.2157)
  line L612 (8.6807, 1.2157) -> (8.4945, 1.0554)
  line L613 (8.4945, 1.0554) -> (8.3487, 0.9383)
  line L614 (8.3487, 0.9383) -> (7.7517, 1.193)
  line L615 (7.7517, 1.193) -> (7.7353, 1.3792)
  line L616 (7.7353, 1.3792) -> (7.7221, 1.6246)
  line L617 (7.7221, 1.6246) -> (7.7191, 1.8662)
  line L618 (7.7191, 1.8662) -> (7.7266, 2.1036)
  line L619 (7.7266, 2.1036) -> (7.7453, 2.3362)
  line L620 (7.7453, 2.3362) -> (7.7759, 2.5635)
  line L621 (7.7759, 2.5635) -> (7.8199, 2.7843)
  line L622 (7.8199, 2.7843) -> (7.8802, 2.997)
  line L623 (7.8802, 2.997) -> (7.919, 3.0989)
  line L624 (7.919, 3.0989) -> (7.9424, 3.2088)
  line L625 (7.9424, 3.2088) -> (7.9552, 3.3246)
  line L626 (7.9552, 3.3246) -> (7.9527, 3.3873)
  line L627 (7.9527, 3.3873) -> (7.9382, 3.4566)
  line L628 (7.9382, 3.4566) -> (7.8576, 3.5626)
  line L629 (7.8576, 3.5626) -> (7.3558, 3.8594)
  line L630 (7.3558, 3.8594) -> (7.2241, 3.8789)
  line L631 (7.2241, 3.8789) -> (7.1564, 3.8582)
  line L632 (7.1564, 3.8582) -> (7.1002, 3.8302)
  line L633 (7.1002, 3.8302) -> (7.0049, 3.7633)
  line L634 (7.0049, 3.7633) -> (6.9198, 3.6898)
  line L635 (6.9198, 3.6898) -> (6.8493, 3.6067)
  line L636 (6.8493, 3.6067) -> (6.692, 3.4514)
  line L637 (6.692, 3.4514) -> (6.5196, 3.3065)
  line L638 (6.5196, 3.3065) -> (6.3352, 3.1701)
  line L639 (6.3352, 3.1701) -> (6.1403, 3.0417)
  line L640 (6.1403, 3.0417) -> (5.936, 2.9207)
  line L641 (5.936, 2.9207) -> (5.7228, 2.807)
  line L642 (5.7228, 2.807) -> (5.5014, 2.7003)
  line L643 (5.5014, 2.7003) -> (5.3303, 2.625)
  line L644 (5.3303, 2.625) -> (4.8195, 3.0255)
  line L645 (4.8195, 3.0255) -> (4.8519, 3.2096)
  line L646 (4.8519, 3.2096) -> (4.9026, 3.4501)
  line L647 (4.9026, 3.4501) -> (4.9623, 3.6842)
  line L648 (4.9623, 3.6842) -> (5.031, 3.9115)
  line L649 (5.031, 3.9115) -> (5.1092, 4.1314)
  line L650 (5.1092, 4.1314) -> (5.1976, 4.343)
  line L651 (5.1976, 4.343) -> (5.2973, 4.545)
  line L652 (5.2973, 4.545) -> (5.4105, 4.7348)
  line L653 (5.4105, 4.7348) -> (5.4744, 4.8231)
  line L654 (5.4744, 4.8231) -> (5.5255, 4.9233)
  line L655 (5.5255, 4.9233) -> (5.5678, 5.0318)
  line L656 (5.5678, 5.0318) -> (5.5816, 5.093)
  line L657 (5.5816, 5.093) -> (5.5855, 5.1637)
  line L658 (5.5855, 5.1637) -> (5.5352, 5.287)
  line L659 (5.5352, 5.287) -> (5.1272, 5.7035)
  line L660 (5.1272, 5.7035) -> (5.0051, 5.7565)
  line L661 (5.0051, 5.7565) -> (4.9343, 5.754)
  line L662 (4.9343, 5.754) -> (4.8728, 5.7415)
  line L663 (4.8728, 5.7415) -> (4.7634, 5.7015)
  line L664 (4.7634, 5.7015) -> (4.6622, 5.6525)
  line L665 (4.6622, 5.6525) -> (4.5726, 5.5905)
  line L666 (4.5726, 5.5905) -> (4.3804, 5.4812)
  line L667 (4.3804, 5.4812) -> (4.1764, 5.3858)
  line L668 (4.1764, 5.3858) -> (3.963, 5.3019)
  line L669 (3.963, 5.3019) -> (3.7416, 5.2283)
  line L670 (3.7416, 5.2283) -> (3.5128, 5.1643)
  line L671 (3.5128, 5.1643) -> (3.2775, 5.1096)
  line L672 (3.2775, 5.1096) -> (3.0361, 5.0639)
  line L673 (3.0361, 5.0639) -> (2.8513, 5.0354)
  line L674 (2.8513, 5.0354) -> (2.4615, 5.5544)
  line L675 (2.4615, 5.5544) -> (2.5405, 5.724)
  line L676 (2.5405, 5.724) -> (2.6517, 5.943)
  line L677 (2.6517, 5.943) -> (2.7699, 6.1538)
  line L678 (2.7699, 6.1538) -> (2.8951, 6.3556)
  line L679 (2.8951, 6.3556) -> (3.0276, 6.5477)
  line L680 (3.0276, 6.5477) -> (3.1678, 6.7292)
  line L681 (3.1678, 6.7292) -> (3.3163, 6.8985)
  line L682 (3.3163, 6.8985) -> (3.4749, 7.0525)
  line L683 (3.4749, 7.0525) -> (3.5594, 7.1213)
  line L684 (3.5594, 7.1213) -> (3.6347, 7.2049)
  line L685 (3.6347, 7.2049) -> (3.7036, 7.2988)
  line L686 (3.7036, 7.2988) -> (3.7328, 7.3543)
  line L687 (3.7328, 7.3543) -> (3.7549, 7.4216)
  line L688 (3.7549, 7.4216) -> (3.7381, 7.5536)
  line L689 (3.7381, 7.5536) -> (3.4519, 8.0616)
  line L690 (3.4519, 8.0616) -> (3.3476, 8.1443)
  line L691 (3.3476, 8.1443) -> (3.2787, 8.1603)
  line L692 (3.2787, 8.1603) -> (3.216, 8.1641)
  line L693 (3.216, 8.1641) -> (3.1, 8.1538)
  line L694 (3.1, 8.1538) -> (2.9895, 8.1327)
  line L695 (2.9895, 8.1327) -> (2.8869, 8.096)
  line L696 (2.8869, 8.096) -> (2.673, 8.0402)
  line L697 (2.673, 8.0402) -> (2.4513, 8.0008)
  line L698 (2.4513, 8.0008) -> (2.2234, 7.975)
  line L699 (2.2234, 7.975) -> (1.9904, 7.9612)
  line L700 (1.9904, 7.9612) -> (1.753, 7.9586)
  line L701 (1.753, 7.9586) -> (1.5115, 7.9666)
  line L702 (1.5115, 7.9666) -> (1.2664, 7.985)
  line L703 (1.2664, 7.985) -> (1.0806, 8.0053)
  line L704 (1.0806, 8.0053) -> (0.8385, 8.6075)
  line L705 (0.8385, 8.6075) -> (0.9586, 8.7508)
  line L706 (0.9586, 8.7508) -> (1.1227, 8.9337)
  line L707 (1.1227, 8.9337) -> (1.2914, 9.1066)
  line L708 (1.2914, 9.1066) -> (1.4646, 9.2691)
  line L709 (1.4646, 9.2691) -> (1.6424, 9.4205)
  line L710 (1.6424, 9.4205) -> (1.8247, 9.5595)
  line L711 (1.8247, 9.5595) -> (2.012, 9.6846)
  line L712 (2.012, 9.6846) -> (2.205, 9.7923)
  line L713 (2.205, 9.7923) -> (2.3045, 9.8369)
  line L714 (2.3045, 9.8369) -> (2.3988, 9.8981)
  line L715 (2.3988, 9.8981) -> (2.4897, 9.9709)
  line L716 (2.4897, 9.9709) -> (2.5322, 10.0171)
  line L717 (2.5322, 10.0171) -> (2.571, 10.0763)
  line L718 (2.571, 10.0763) -> (2.589, 10.2082)
  line L719 (2.589, 10.2082) -> (2.444, 10.7729)
  line L720 (10.6887, 11.9736) -> (4.3034, 11.2009)
  line L721 (4.3034, 11.2009) -> (3.9458, 10.6765)
  line L722 (3.9458, 10.6765) -> (4.1371, 10.064)
  line L723 (4.1371, 10.064) -> (4.3688, 9.4655)
  line L724 (4.3688, 9.4655) -> (4.6397, 8.8838)
  line L725 (4.6397, 8.8838) -> (4.9487, 8.3214)
  line L726 (4.9487, 8.3214) -> (5.2943, 7.7807)
  line L727 (5.2943, 7.7807) -> (5.6752, 7.2642)
  line L728 (5.6752, 7.2642) -> (6.0896, 6.7742)
  line L729 (6.0896, 6.7742) -> (6.5356, 6.3128)
  line L730 (6.5356, 6.3128) -> (7.0113, 5.8821)
  line L731 (7.0113, 5.8821) -> (7.5145, 5.484)
  line L732 (7.5145, 5.484) -> (8.0432, 5.1202)
  line L733 (8.0432, 5.1202) -> (8.5948, 4.7923)
  line L734 (8.5948, 4.7923) -> (9.167, 4.5019)
  line L735 (9.167, 4.5019) -> (9.7573, 4.2501)
  line L736 (9.7573, 4.2501) -> (10.363, 4.0381)
  line L737 (10.363, 4.0381) -> (10.9815, 3.8669)
  line L738 (10.9815, 3.8669) -> (11.6099, 3.7372)
  line L739 (11.6099, 3.7372) -> (12.2456, 3.6495)
  line L740 (12.2456, 3.6495) -> (12.8858, 3.6043)
  line L741 (12.8858, 3.6043) -> (13.5275, 3.6017)
  line L742 (13.5275, 3.6017) -> (14.1679, 3.6418)
  line L743 (14.1679, 3.6418) -> (14.8043, 3.7244)
  line L744 (14.8043, 3.7244) -> (15.4338, 3.8491)
  line L745 (15.4338, 3.8491) -> (16.0536, 4.0153)
  line L746 (16.0536, 4.0153) -> (16.661, 4.2225)
  line L747 (16.661, 4.2225) -> (17.2532, 4.4695)
  line L748 (17.2532, 4.4695) -> (17.8278, 4.7554)
  line L749 (17.8278, 4.7554) -> (17.9587, 5.3764)
  line L750 (17.9587, 5.3764) -> (14.0969, 10.5199)
  line L751 (14.0969, 10.5199) -> (13.2632, 10.8348)
  line L752 (13.2632, 10.8348) -> (12.9342, 10.8549)
  line L753 (12.9342, 10.8549) -> (12.6109, 10.9197)
  line L754 (12.6109, 10.9197) -> (12.2995, 11.028)
  line L755 (12.2995, 11.028) -> (12.0058, 11.1777)
  line L756 (12.0058, 11.1777) -> (11.7353, 11.3662)
  line L757 (11.7353, 11.3662) -> (11.493, 11.5898)
  line L758 (11.493, 11.5898) -> (10.6887, 11.9736)
  line L759 (15.6248, 11.667) -> (19.4866, 6.5236)
  line L760 (19.4866, 6.5236) -> (20.1195, 6.476)
  line L761 (20.1195, 6.476) -> (20.5543, 6.948)
  line L762 (20.5543, 6.948) -> (20.9568, 7.4479)
  line L763 (20.9568, 7.4479) -> (21.3251, 7.9733)
  line L764 (21.3251, 7.9733) -> (21.6577, 8.5221)
  line L765 (21.6577, 8.5221) -> (21.9531, 9.0918)
  line L766 (21.9531, 9.0918) -> (22.2099, 9.6799)
  line L767 (22.2099, 9.6799) -> (22.4271, 10.2837)
  line L768 (22.4271, 10.2837) -> (22.6037, 10.9007)
  line L769 (22.6037, 10.9007) -> (22.7389, 11.528)
  line L770 (22.7389, 11.528) -> (22.832, 12.1629)
  line L771 (22.832, 12.1629) -> (22.8828, 12.8026)
  line L772 (22.8828, 12.8026) -> (22.8909, 13.4443)
  line L773 (22.8909, 13.4443) -> (22.8563, 14.0851)
  line L774 (22.8563, 14.0851) -> (22.7792, 14.7222)
  line L775 (22.7792, 14.7222) -> (22.6599, 15.3527)
  line L776 (22.6599, 15.3527) -> (22.499, 15.9739)
  line L777 (22.499, 15.9739) -> (22.2971, 16.5831)
  line L778 (22.2971, 16.5831) -> (22.0552, 17.1774)
  line L779 (22.0552, 17.1774) -> (21.7743, 17.7544)
  line L780 (21.7743, 17.7544) -> (21.4557, 18.3114)
  line L781 (21.4557, 18.3114) -> (21.1007, 18.846)
  line L782 (21.1007, 18.846) -> (20.711, 19.3559)
  line L783 (20.711, 19.3559) -> (20.2883, 19.8387)
  line L784 (20.2883, 19.8387) -> (19.8344, 20.2923)
  line L785 (19.8344, 20.2923) -> (19.3513, 20.7147)
  line L786 (19.3513, 20.7147) -> (18.8412, 21.1041)
  line L787 (18.8412, 21.1041) -> (18.3064, 21.4588)
  line L788 (18.3064, 21.4588) -> (17.7031, 21.2616)
  line L789 (17.7031, 21.2616) -> (15.1796, 15.3455)
  line L790 (15.1796, 15.3455) -> (15.3238, 14.4661)
  line L791 (15.3238, 14.4661) -> (15.4709, 14.171)
  line L792 (15.4709, 14.171) -> (15.5764, 13.8587)
  line L793 (15.5764, 13.8587) -> (15.6383, 13.5348)
  line L794 (15.6383, 13.5348) -> (15.6555, 13.2056)
  line L795 (15.6555, 13.2056) -> (15.6275, 12.8771)
  line L796 (15.6275, 12.8771) -> (15.555, 12.5555)
  line L797 (15.555, 12.5555) -> (15.6248, 11.667)
  line L798 (13.4223, 16.0951) -> (15.9457, 22.0112)
  line L799 (15.9457, 22.0112) -> (15.6704, 22.5831)
  line L800 (15.6704, 22.5831) -> (15.0442, 22.7237)
  line L801 (15.0442, 22.7237) -> (14.4102, 22.8223)
  line L802 (14.4102, 22.8223) -> (13.7709, 22.8786)
  line L803 (13.7709, 22.8786) -> (13.1293, 22.8922)
  line L804 (13.1293, 22.8922) -> (12.4883, 22.8632)
  line L805 (12.4883, 22.8632) -> (11.8506, 22.7916)
  line L806 (11.8506, 22.7916) -> (11.219, 22.6777)
  line L807 (11.219, 22.6777) -> (10.5964, 22.5222)
  line L808 (10.5964, 22.5222) -> (9.9856, 22.3256)
  line L809 (9.9856, 22.3256) -> (9.3891, 22.0888)
  line L810 (9.3891, 22.0888) -> (8.8098, 21.8129)
  line L811 (8.8098, 21.8129) -> (8.25, 21.4991)
  line L812 (8.25, 21.4991) -> (7.7124, 21.1487)
  line L813 (7.7124, 21.1487) -> (7.1992, 20.7634)
  line L814 (7.1992, 20.7634) -> (6.7128, 20.3449)
  line L815 (6.7128, 20.3449) -> (6.2553, 19.8949)
  line L816 (6.2553, 19.8949) -> (5.8286, 19.4155)
  line L817 (5.8286, 19.4155) -> (5.4349, 18.9088)
  line L818 (5.4349, 18.9088) -> (5.0756, 18.377)
  line L819 (5.0756, 18.377) -> (4.7526, 17.8226)
  line L820 (4.7526, 17.8226) -> (4.4671, 17.2479)
  line L821 (4.4671, 17.2479) -> (4.2204, 16.6555)
  line L822 (4.2204, 16.6555) -> (4.0136, 16.048)
  line L823 (4.0136, 16.048) -> (3.8477, 15.4281)
  line L824 (3.8477, 15.4281) -> (3.7234, 14.7985)
  line L825 (3.7234, 14.7985) -> (3.6412, 14.1621)
  line L826 (3.6412, 14.1621) -> (3.6015, 13.5216)
  line L827 (3.6015, 13.5216) -> (4.0739, 13.0976)
  line L828 (4.0739, 13.0976) -> (10.4591, 13.8703)
  line L829 (10.4591, 13.8703) -> (11.1487, 14.4349)
  line L830 (11.1487, 14.4349) -> (11.3306, 14.7098)
  line L831 (11.3306, 14.7098) -> (11.5484, 14.9574)
  line L832 (11.5484, 14.9574) -> (11.7979, 15.1729)
  line L833 (11.7979, 15.1729) -> (12.0745, 15.3524)
  line L834 (12.0745, 15.3524) -> (12.3729, 15.4924)
  line L835 (12.3729, 15.4924) -> (12.6877, 15.5904)
  line L836 (12.6877, 15.5904) -> (13.4223, 16.0951)
  circle A0 centre (13.2452, 13.2452) radius 0.5
  line L837 (8.8302, 13.2452) -> (17.6603, 13.2452)
  line L838 (13.2452, 8.8302) -> (13.2452, 17.6603)
  constraints: 1678 end point, 1 centre point
extrude "Выдавливание1" add sketch "a" along normal blind 5
sketch "Эскиз4" plane through (0, 0, 5) normal (0, 0, 1) x (1, 0, 0)
  line L0 (12.6362, 11.4749) -> (15.1152, 13.3362)
  line L1 (15.1152, 13.3362) -> (13.8543, 15.0156)
  line L2 (13.8543, 15.0156) -> (11.3753, 13.1543)
  line L3 (11.3753, 13.1543) -> (12.6362, 11.4749)
  circle A0 centre (13.2452, 13.2452) radius 0.5 projected
  line L4 (12.6362, 11.4749) -> (13.8543, 15.0156) construction
  line L5 (15.1152, 13.3362) -> (11.3753, 13.1543) construction
  line L6 (11.7979, 15.1729) -> (11.5484, 14.9574) projected
  line L7 (11.7979, 15.1729) -> (12.6148, 14.0849)
  circle A1 centre (13.2452, 13.2452) radius 0.5 projected
  circle A2 centre (13.2452, 13.2452) radius 1.55
  line L8 (12.1977, 15.4731) -> (13.0146, 14.3851)
  line L9 (13.0146, 14.3851) -> (12.215, 13.7847)
  line L10 (12.215, 13.7847) -> (11.3981, 14.8727)
  line L11 (11.3981, 14.8727) -> (12.1977, 15.4731)
  line L12 (12.1977, 15.4731) -> (12.215, 13.7847) construction
  line L13 (13.0146, 14.3851) -> (11.3981, 14.8727) construction
  point P0 (0, 0)
  point P1 (12.2063, 14.6289)
  point P2 (11.9645, 14.1183)
  point P3 (12.9639, 11.721)
  point P4 (14.7875, 13.0902)
  point P5 (12.7642, 14.7187)
  dimension "d2" = 3.1
  dimension "d3" = 2.1
  dimension "d4" = 1
  constraints: 26 end point, 6 midpoint, 4 parallel, 3 perpendicular, 1 centre point, 1 coincident, 1 collinear, 1 tangent
  measures "d2" diameter of A2
  measures "d3" distance of L0.end L1.end
  measures "d4" distance between parallel lines of L8 L10
extrude "Выдавливание2" cut sketch "Эскиз4" against normal through all contours A2 L2 L0 | A2 L10 L2 | L10 A2 L7 L2 | L10 L11 L7 A2 | L7 A2 L8 L2 | L7 L11 L8 A2 | L2 L8 A2 | A0
